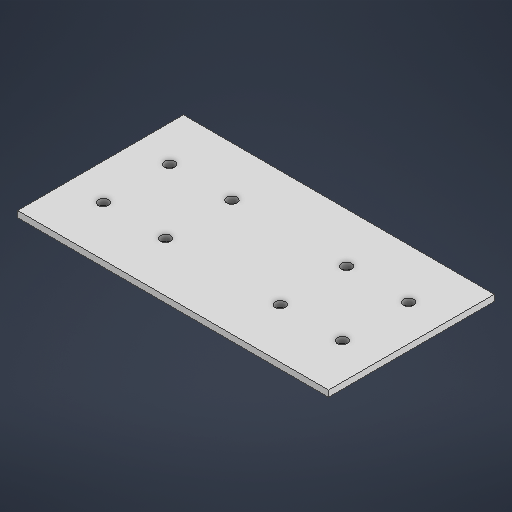
# Autodesk Inventor part: X Axis Base Plate
Saved by Autodesk Inventor 2025.1 (Build 291241000, 241)
## iProperties
Created: 2024-11-10
Part Number: X Axis Base Plate
Material: Generic
Document SubType Name: Modeling
Designer: jerem
Density: 1 g/cm^3
Appearance: Default
Author: jerem
Autodesk Inventor part; units mm, degrees
ref_plane "YZ Plane" through (0, 0, 0) normal (1, 0, 0) x (0, 1, 0)
ref_plane "XZ Plane" through (0, 0, 0) normal (0, 1, 0) x (-1, 0, 0)
ref_plane "XY Plane" through (0, 0, 0) normal (0, 0, 1) x (1, 0, 0)
sketch "Sketch1" plane through (0, 0, 0) normal (0, 1, 0) x (-1, 0, 0)
  line L0 (-75, -40) -> (75, -40)
  line L1 (75, -40) -> (75, 40)
  line L2 (75, 40) -> (-75, 40)
  line L3 (-75, 40) -> (-75, -40)
  line L4 (-75, -40) -> (75, 40) construction
  line L5 (75, -40) -> (-75, 40) construction
  circle A0 centre (-57.65, 16) radius 2.5
  circle A1 centre (-27.65, 16) radius 2.5
  line L6 (-57.65, 16) -> (-27.65, 16) construction
  circle A2 centre (-57.65, -16) radius 2.5
  circle A3 centre (-27.65, -16) radius 2.5
  line L7 (-57.65, -16) -> (-27.65, -16) construction
  line L8 (-42.65, 16) -> (-42.65, -16) construction
  line L9 (27.65, -16) -> (57.65, -16) construction
  circle A4 centre (57.65, -16) radius 2.5
  circle A5 centre (27.65, -16) radius 2.5
  line L10 (27.65, 16) -> (57.65, 16) construction
  circle A6 centre (57.65, 16) radius 2.5
  circle A7 centre (27.65, 16) radius 2.5
  line L11 (42.65, 16) -> (42.65, -16) construction
  line L12 (42.65, 0) -> (0, 0) construction
  line L13 (0, 0) -> (-42.65, 0) construction
  line L14 (20, -22) -> (65.3, -22) construction
  line L15 (65.3, -22) -> (65.3, 22) construction
  line L16 (65.3, 22) -> (20, 22) construction
  line L17 (20, 22) -> (20, -22) construction
  line L18 (20, -22) -> (65.3, 22) construction
  line L19 (65.3, -22) -> (20, 22) construction
  line L20 (-65.3, -22) -> (-20, -22) construction
  line L21 (-20, -22) -> (-20, 22) construction
  line L22 (-20, 22) -> (-65.3, 22) construction
  line L23 (-65.3, 22) -> (-65.3, -22) construction
  line L24 (-65.3, -22) -> (-20, 22) construction
  line L25 (-20, -22) -> (-65.3, 22) construction
  dimension "d0" = 150
  dimension "d1" = 80
  dimension "d2" = 5
  dimension "d3" = 5
  dimension "d4" = 30
  dimension "d5" = 5
  dimension "d6" = 5
  dimension "d7" = 30
  dimension "d8" = 32
  dimension "d9" = 5
  dimension "d10" = 5
  dimension "d11" = 30
  dimension "d12" = 5
  dimension "d13" = 5
  dimension "d14" = 30
  dimension "d15" = 32
  dimension "d16" = 45.3
  dimension "d17" = 44
  dimension "d18" = 45.3
  dimension "d19" = 44
  dimension "d20" = 40
  constraints: 52 end point, 12 midpoint, 8 centre point, 6 horizontal, 6 parallel, 6 perpendicular, 1 collinear
  measures "d0" distance of L2.end L1.end
  measures "d1" distance of L1.end L0.end
  measures "d2" diameter of A0
  measures "d3" diameter of A1
  measures "d4" distance of L6.start L6.end
  measures "d5" diameter of A2
  measures "d6" diameter of A3
  measures "d7" distance of L7.start L7.end
  measures "d8" distance between parallel lines of L6 L7
  measures "d9" diameter of A7
  measures "d10" diameter of A6
  measures "d11" distance of L10.start L10.end
  measures "d12" diameter of A5
  measures "d13" diameter of A4
  measures "d14" distance of L9.start L9.end
  measures "d15" distance between parallel lines of L10 L9
  measures "d16" distance of L16.end L15.end
  measures "d17" distance of L15.end L14.end
  measures "d18" distance of L22.end L21.end
  measures "d19" distance of L21.end L20.end
  measures "d20" distance between parallel lines of L21 L17
extrude "Extrusion1" add sketch "Sketch1" along normal blind 3
equation "\"d3\" = d2"
equation "\"d6\" = d5"
equation "\"d7\" = d4"
equation "\"d10\" = d9"
equation "\"d11\" = d4"
equation "\"d13\" = d12"
equation "\"d14\" = d4"
body "Solid1"
